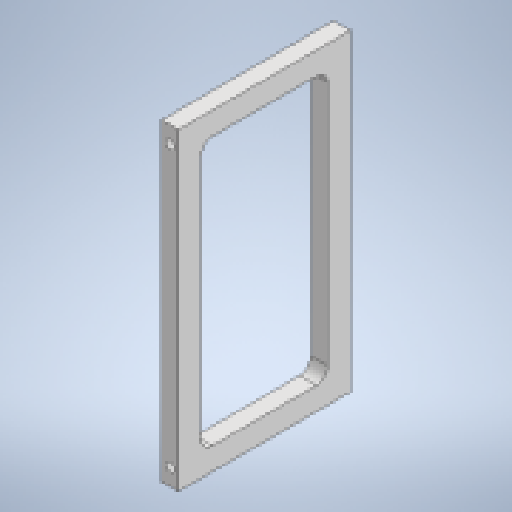
# Autodesk Inventor part: kosinosita
Saved by Autodesk Inventor 2025.1 (Build 291241000, 241)
## iProperties
Created: 2024-09-01
Part Number: kosinosita
Material: 一般
Document SubType Name: Modeling
Designer: right
Density: 1 g/cm^3
Appearance: 既定
Author: right
Autodesk Inventor part; units mm, degrees
ref_plane "YZ Plane" through (0, 0, 0) normal (1, 0, 0) x (0, 1, 0)
ref_plane "XZ Plane" through (0, 0, 0) normal (0, 1, 0) x (-1, 0, 0)
sketch "スケッチ1" plane through (0, 0, 0) normal (0, 0, 1) x (1, 0, 0)
  circle A0 centre (23.0793, 24.731) radius 1.1 projected
  circle A1 centre (23.0793, -24.731) radius 1.1 projected
  line L0 (24.5793, 27.731) -> (21.5793, 27.731)
  line L1 (21.5793, 27.731) -> (21.5793, -27.731)
  line L2 (21.5793, -27.731) -> (24.5793, -27.731)
  line L3 (24.5793, -27.731) -> (24.5793, 27.731)
  point P0 (0, 0)
  point P1 (23.0793, 27.731)
  dimension "d0" = 3
  dimension "d1" = 3
  dimension "d2" = 3
  constraints: 8 end point, 2 parallel, 1 horizontal, 1 midpoint, 1 perpendicular, 1 vertical alignment
  measures "d0" distance of L2.end L1.end
  measures "d1" distance from line of L0 A0.centre
  measures "d2" distance from line of A1.centre L2
ref_plane "作業平面1" through (-53.6786, -65.4442, 30.5) normal (0, 0, -1) x (0.7071068, 0.7071068, 0)
extrude "押し出し1" add sketch "スケッチ1" along normal up to surface (30.5 mm away) contours A0 | A1 | L3 L2 L1 L0
sketch "スケッチ2" plane through (0, 0, 0) normal (0, 0, -1) x (-1, 0, 0)
  circle A0 centre (-23.0793, 24.731) radius 1.1 projected
  circle A1 centre (-23.0793, -24.731) radius 1.1 projected
  point P0 (0, 0)
  constraints: 2 coincident
hole "穴1" at (23.0793, 24.731, 0) at (23.0793, -24.731, 0) direction (0, 0, 1) diameter 1.567 end through all thread size "M2x0.4" class "6H" standard "ISO Metric profile"
sketch "スケッチ3" plane through (24.5793, -27.731, 0) normal (1, 0, 0) x (0, 0, -1)
  line L0 (-30.5, 0) -> (-30.5, 55.4619) projected
  line L1 (0, 0) -> (-30.5, 0) projected
  line L2 (0, 0) -> (0, 55.4619) projected
  line L3 (0, 55.4619) -> (-30.5, 55.4619) projected
  line L4 (-4, 51.4619) -> (-4, 4)
  line L5 (-4, 4) -> (-26.5, 4)
  line L6 (-26.5, 4) -> (-26.5, 51.4619)
  line L7 (-26.5, 51.4619) -> (-4, 51.4619)
  point P0 (0, 27.731)
  dimension "d12" = 4
  constraints: 8 end point, 3 other
  measures "d12" distance between parallel lines of L3 L7
extrude "押し出し2" cut sketch "スケッチ3" against normal through all contours L4 L5 L6 L7
fillet "フィレット1" radius 2 4 edges at (23.0793, 23.731, 26.5) (23.0793, 23.731, 4) (23.0793, -23.731, 26.5) (23.0793, -23.731, 4)
sketch "スケッチ4" plane through (24.5793, -27.731, 0) normal (1, 0, 0) x (0, 0, -1)
  line L0 (0, 53.2454) -> (0, 51.6784) construction
  line L1 (0, 3.7835) -> (0, 2.2165) construction
  line L2 (-30.5, 4.1) -> (-30.5, 1.9) construction
  line L3 (-30.5, 51.6784) -> (-30.5, 53.2454) construction
  circle A0 centre (-31.5, 52.4619) radius 1.1
  line L4 (0, 27.731) -> (-30.5, 27.731) construction
  line L5 (-30.5, 0) -> (-30.5, 55.4619) construction
  line L6 (-15.25, 27.731) -> (-15.25, 0) construction
  line L7 (0, 0) -> (-30.5, 0) construction
  circle A1 centre (-31.5, 3) radius 1.1
  circle A2 centre (1, 52.4619) radius 1.1
  circle A3 centre (1, 3) radius 1.1
  point P0 (-30.5, 52.4619)
  dimension "d16" = 2.2
  dimension "d17" = 1
  constraints: 4 centre point, 4 end point, 4 midpoint, 3 symmetric about line, 1 horizontal alignment, 3 other
  measures "d16" diameter of A0
  measures "d17" distance from line of L3 A0.centre
extrude "押し出し3" cut sketch "スケッチ4" against normal through all
equation "\"d2\" = d1"
